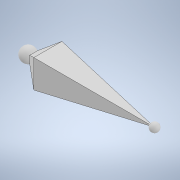
# Autodesk Inventor part: Bone
Saved by Autodesk Inventor 2021 (Build 250183000, 183)
## iProperties
Created: 2021-10-25
Part Number: Bone
Material: 一般
Document SubType Name: Modeling
Designer: RTon
Density: 1 g/cm^3
Appearance: 預設
Author: RTon
Autodesk Inventor part; units mm, degrees
ref_plane "YZ Plane" through (0, 0, 0) normal (1, 0, 0) x (0, 1, 0)
ref_plane "XZ Plane" through (0, 0, 0) normal (0, 1, 0) x (-1, 0, 0)
ref_plane "XY Plane" through (0, 0, 0) normal (0, 0, 1) x (1, 0, 0)
sketch "草圖3" plane through (0, 0, 0) normal (0, 1, 0) x (-1, 0, 0)
  line L0 (0, 50) -> (-450, 50)
  line L1 (-450, 50) -> (-450, -50)
  line L2 (-450, -50) -> (0, -50)
  line L3 (0, -50) -> (0, 50)
  point P0 (0, 0)
  point P1 (0, 0)
  dimension "d17" = 100
  dimension "d18" = 450
  constraints: 8 end point, 2 midpoint, 2 parallel, 1 coincident, 1 horizontal, 1 perpendicular
  measures "d17" distance of L0.end L1.end
  measures "d18" distance of L1.end L2.end
extrude "擠出3" add sketch "草圖3" along normal mid plane 100
chamfer "倒角4" distance 50 distance2 70 1 edges at (0, 0, 50) measured on face at (0, -16.6667, -16.6667)
chamfer "倒角5" distance 70 distance2 50 1 edges at (0, -50, -25) measured on face at (173.3333, -50, -16.6667)
chamfer "倒角6" distance 70 distance2 50 1 edges at (0, 25, -50) measured on face at (173.3333, 16.6667, -50)
chamfer "倒角8" distance 50 distance2 380 1 edges at (450, 0, -50) measured on face at (450, 16.6667, -16.6667)
chamfer "倒角9" distance 380 distance2 50 1 edges at (450, 50, 25) measured on face at (196.6667, 50, 0)
chamfer "倒角10" distance 50 distance2 380 1 edges at (450, -25, 50) measured on face at (450, -33.3333, 33.3333)
sketch "草圖4" plane through (0, 0, 0) normal (0, 0, 1) x (1, 0, 0)
  line L0 (450, -50) -> (70, -50) projected
  line L1 (450, 0) -> (70, 50) projected
  line L2 (70, -50) -> (450, 0)
  line L3 (450, 0) -> (450, -50) projected
  line L4 (450, 0) -> (450, -50)
  line L5 (450, -50) -> (70, -50)
  point P0 (0, 0)
  point P1 (70, 50)
  point P2 (170, -50)
  point P3 (170, 50)
  constraints: 6 end point, 1 collinear, 1 perpendicular, 1 other
extrude "擠出4" cut sketch "草圖4" along normal mid plane 100
sketch "草圖5" plane through (0, 0, 0) normal (0, 0, 1) x (1, 0, 0)
  line L0 (70, -50) -> (0, 0) projected
  line L1 (0, 50) -> (0, 0) projected
  line L2 (0, 0) -> (0, 50)
  line L3 (70, 50) -> (70, -50) projected
  line L4 (0, 50) -> (70, 50)
  line L5 (70, 50) -> (0, 0)
  constraints: 6 end point, 1 perpendicular, 1 vertical
extrude "擠出5" cut sketch "草圖5" along normal mid plane 100 contours L1 L4 L5
sketch "草圖6" plane through (0, 0, 0) normal (1, 0, 0) x (0, 1, 0)
  circle A0 centre (0, 0) radius 25
  line L0 (0, 25) -> (0, -25)
  point P0 (0, 0)
  dimension "d46" = 50
  constraints: 2 end point, 2 point on circle, 1 centre point, 1 coincident, 1 vertical
  measures "d46" diameter of A0
revolve "迴轉1" add sketch "草圖6" angle 360 about axis through (0, 0, 25) along (0, 0, -1) picked at (-8.8525, -4.4917) contours L0 A0
sketch "草圖7" plane through (0, 0, 0) normal (0, 1, 0) x (-1, 0, 0)
  line L0 (-450, 0) -> (-70, -50) projected
  circle A0 centre (-450, 0) radius 15
  line L1 (-450, 15) -> (-450, -15)
  point P0 (0, 0)
  dimension "d48" = 30
  constraints: 2 end point, 2 point on circle, 1 centre point, 1 vertical
  measures "d48" diameter of A0
revolve "迴轉2" add sketch "草圖7" angle 360 about axis through (450, 0, 15) along (0, 0, -1) contours L1 A0
